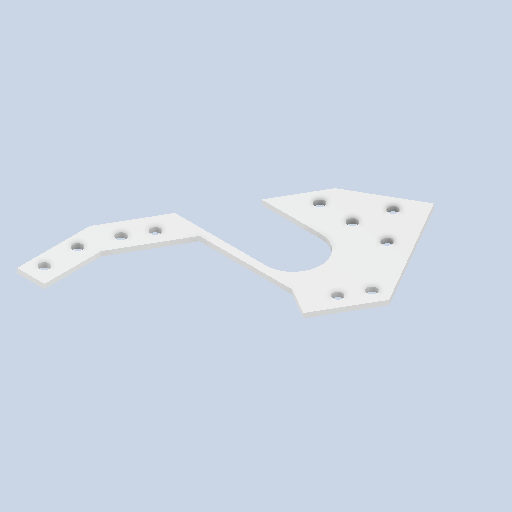
# Autodesk Inventor part: base_cover
Saved by Autodesk Inventor 2024.1 (Build 281209000, 209)
## iProperties
Created: 2025-01-17
Part Number: base_cover
Material: アルミニウム 6061
Document SubType Name: Sheet Metal
Designer: hibik
Density: 2.7 g/cm^3
Sheet Metal Rule: Default_mm
Appearance: アルミニウム - フラット
Author: hibik
Autodesk Inventor part; units mm, degrees
ref_plane "YZ Plane" through (0, 0, 0) normal (1, 0, 0) x (0, 1, 0)
ref_plane "XZ Plane" through (0, 0, 0) normal (0, 1, 0) x (-1, 0, 0)
ref_plane "XY Plane" through (0, 0, 0) normal (0, 0, 1) x (1, 0, 0)
sketch "スケッチ2" plane through (0, 0, 0) normal (0, 1, 0) x (-1, 0, 0)
  line L0 (0, 0) -> (40, 0)
  line L1 (40, 0) -> (40, -23.7735)
  line L2 (-30, -51.9615) -> (0, 0)
  line L3 (-30, -51.9615) -> (-10, -86.6025)
  line L4 (-10, -86.6025) -> (10.5885, -74.7158)
  line L5 (10.5885, -74.7158) -> (40, -23.7735)
  line L6 (-30, -51.9615) -> (-36.3397, -48.3013) construction
  line L7 (30, 0) -> (30, -18) construction
  line L8 (30, -18) -> (40, -23.7735) construction
  dimension "d0" = 60
  dimension "d1" = 60
  dimension "d2" = 40
  dimension "d3" = 60
  dimension "d4" = 18
  dimension "d5" = 30
  dimension "d6" = 60
  measures "d0" angle of L0 L2
  measures "d1" angle of L2 L3
  measures "d2" distance of L0.start L0.end
  measures "d3" distance from line of L0.start L6
  measures "d4" distance of L7.start L7.end
  measures "d5" distance from line of L0.start L7
  measures "d6" angle of L7 L8
extrude "プレート1" add sketch "スケッチ2" along normal blind 1.5
sketch "スケッチ3" plane through (0, 1.5, 0) normal (0, 1, 0) x (1, 0, 0)
  line L0 (-10.5885, 74.7158) -> (-40, 23.7735) projected
  line L1 (-31.7863, 38) -> (10.9697, 38)
  line L2 (10.9697, 38) -> (19.1969, 33.25)
  line L3 (0, 0) -> (30, 51.9615) projected
  line L4 (30, 51.9615) -> (0, 0) projected
  line L5 (0, 0) -> (-40, 0) projected
  circle A0 centre (0, 50.5) radius 12.5 construction
  circle A1 centre (0, 50.5) radius 1.5
  circle A2 centre (0, 50.5) radius 10.5 construction
  circle A3 centre (5.9346, 70.644) radius 10.5 construction
  circle A4 centre (5.9346, 70.644) radius 11.5 construction
  line L6 (10, 86.6025) -> (30, 51.9615) projected
  circle A5 centre (5.9346, 70.644) radius 1.5
  line L7 (-30, 0) -> (-30, 18)
  line L8 (-30, 18) -> (-18.453, 38)
  line L9 (-40, 23.7735) -> (-10.5885, 74.7158) projected
  line L10 (-40, 23.7735) -> (-40, 0) projected
  line L11 (-40, 23.7735) -> (-30, 18)
  line L12 (-31, 0) -> (-31, 18.5774)
  line L13 (-19.209, 39) -> (-31, 18.5774)
  line L14 (-19.209, 39) -> (11.2376, 39)
  line L15 (11.2376, 39) -> (19.6969, 34.116)
  circle A6 centre (0, 50.5) radius 9
  line L16 (-29.7656, 59.5) -> (9, 59.5)
  line L17 (9, 59.5) -> (9, 41.5) construction
  line L18 (9, 41.5) -> (-29.7656, 41.5)
  line L19 (-29.7656, 41.5) -> (-29.7656, 59.5)
  line L20 (-29.7656, 41.5) -> (-19.3733, 59.5)
  line L21 (0, 59.5) -> (0, 41.5)
  dimension "d8" = 38
  dimension "d9" = 9.5
  dimension "d10" = 25
  dimension "d11" = 3
  dimension "d14" = 21
  dimension "d15" = 21
  dimension "d16" = 23
  dimension "d17" = 3
  dimension "d18" = 30
  dimension "d19" = 18
  dimension "d21" = 1
  dimension "d22" = 1
  dimension "d23" = 1
  dimension "d24" = 18
  constraints: 30 end point, 12 point on line, 7 centre point, 6 parallel, 6 tangent, 5 coincident, 3 horizontal, 2 perpendicular, 2 point on circle, 1 vertical, 1 vertical alignment
  measures "d8" distance between parallel lines of L5 L1
  measures "d9" distance from line of L1.end L3
  measures "d10" diameter of A0
  measures "d11" diameter of A1
  measures "d14" diameter of A2
  measures "d15" diameter of A3
  measures "d16" diameter of A4
  measures "d17" diameter of A5
  measures "d18" distance from line of L3.start L7
  measures "d19" distance of L7.start L7.end
  measures "d21" distance between parallel lines of L7 L12
  measures "d22" distance between parallel lines of L1 L14
  measures "d23" distance between parallel lines of L15 L2
  measures "d24" diameter of A6
extrude "切り取り1" cut sketch "スケッチ3" against normal blind 1.5 contours L16 A6 L18 L0 | L21 A1 A6 | A6 L21 A1 | L21 A1 | A1 L21 | L13 L14 L15 L3 L2 L1 | L1 L8 L11 L13 | L11 L7 L5 L12 | L1 L2 L3 L5 L7 L8
sketch "スケッチ4" plane through (0, 1.5, 0) normal (0, 1, 0) x (1, 0, 0)
  circle A0 centre (5.1388, 78.0224) radius 1.6 projected
  line L0 (14.0853, 64.5965) -> (11.5853, 60.2663) projected
  circle A1 centre (13.1994, 68.061) radius 1.6 projected
  circle A2 centre (-36, 15.8638) radius 1.6 projected
  circle A3 centre (-36, 5) radius 1.6 projected
  circle A4 centre (20.4199, 44.6683) radius 1.6 projected
  circle A5 centre (24.5152, 51.7615) radius 1.6 projected
  circle A6 centre (-27.8315, 33.15) radius 1.6 projected
  circle A7 centre (-31.9338, 26.0447) radius 1.6 projected
  circle A8 centre (-8.7282, 67.9379) radius 1.6 projected
  circle A9 centre (1.9592, 67.9379) radius 1.6 projected
  point P0 (0, 0)
extrude "切り取り2" cut sketch "スケッチ4" against normal blind 1.5
equation "\"d1\" = d0"
equation "\"d12\" = Thickness"
equation "\"d25\" = Thickness"
equation "\"d7\" = Thickness"
equation "\"BendRadius\" = Thickness"
equation "\"BendReliefWidth\" = Thickness"
equation "\"BendReliefDepth\" = 0.5 * Thickness"
equation "\"CornerReliefSize\" = 4 * Thickness"
equation "\"MinimumRemnant\" = 2 * Thickness"
equation "\"TransitionRadius\" = BendRadius"
equation "\"JacobiRadiusSize\" = BendRadius"
equation "\"GapSize\" = Thickness"
equation "\"Thickness\" = 1.5"
